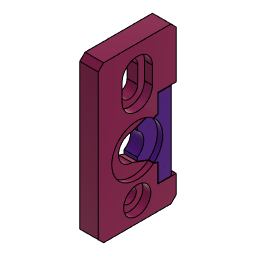
Rod_Holder_Hevo (Autodesk Fusion 360 design; units mm, degrees)
Autodesk Fusion 360 part; units mm, degrees
sketch "Sketch1" plane through (0, 0, 0) normal (1, 0, 0) x (0, 1, 0)
  circle A0 centre (0, 0) radius 5.1
  line L0 (-14.75, 35) -> (14.75, 35)
  line L1 (14.75, 35) -> (14.75, -24)
  line L2 (14.75, -24) -> (-14.75, -24)
  line L3 (-14.75, -24) -> (-14.75, 35)
  line L4 (0, 35) -> (0, -24)
  circle A1 centre (0, 25) radius 3.2
  circle A2 centre (0, 18.4) radius 3.15
  line L5 (0, 18.4) -> (3.15, 18.4) construction
  line L6 (0, 18.4) -> (-3.15, 18.4) construction
  line L7 (-3.15, 18.4) -> (-3.1999, 24.9757)
  line L8 (3.15, 18.4) -> (3.1999, 24.9757)
  arc A3 (5.75, 25) -> (-5.75, 25) centre (0, 25) ccw
  arc A4 (-5.75, 18.4) -> (5.75, 18.4) centre (0, 18.4) ccw
  line L9 (5.75, 18.4) -> (5.75, 25)
  line L10 (-5.75, 25) -> (-5.75, 18.4)
  circle A5 centre (0, -16.5) radius 2.65
  circle A6 centre (0, -16.5) radius 5.15
  line L11 (0, 5.1) -> (7.75, 8)
  line L12 (7.75, 8) -> (7.75, 15)
  line L13 (7.75, 15) -> (14.75, 15)
  line L14 (20, 0) -> (2.5, 0)
  line L15 (0, -5.1) -> (7.75, -8)
  line L16 (7.75, -8) -> (7.75, -15)
  line L17 (7.75, -15) -> (14.75, -15)
  dimension "d1" = 10.2
  dimension "d2" = 29.5
  dimension "d3" = 6.4
  dimension "d4" = 10
  dimension "d5" = 35
  dimension "d6" = 24
  dimension "d7" = 6.3
  dimension "d8" = 6.6
  dimension "d9" = 5.75
  dimension "d10" = 5.75
  dimension "d11" = 5.3
  dimension "d12" = 10.3
  dimension "d13" = 7.5
  dimension "d14" = 7
  dimension "d15" = 7
  dimension "d16" = 15
  constraint coincident A0.centre origin
  constraint horizontal L0
  constraint vertical L1
  constraint horizontal L2
  constraint vertical L3
  constraint midpoint L0 L4.start
  constraint midpoint L2 L4.end
  constraint coincident A0.centre L4
  constraint coincident L4 A1.centre
  constraint coincident L4 A2.centre
  constraint coincident A2.centre L5.start
  constraint coincident A2 L5.end
  constraint perpendicular L4 L5
  constraint coincident A2 L6.end
  constraint perpendicular L4 L6
  constraint coincident A1 L7.end
  constraint tangent A1 L7
  constraint coincident A1 L8.end
  constraint tangent A1 L8
  constraint coincident A1.centre A3.centre
  constraint tangent A3 L9
  constraint tangent A3 L10
  constraint vertical L9
  constraint vertical L10
  constraint coincident L4 A5.centre
  constraint concentric A5 A6
  constraint coincident L4 L11.start
  constraint coincident A0 L11.start
  constraint parallel L4 L12
  constraint coincident L1 L13.end
  constraint perpendicular L1 L13
  constraint symmetric L11.start L14 L15.start
  constraint symmetric L11.end L14 L15.end
  constraint symmetric L12.end L14 L16.end
  constraint symmetric L13.end L14 L17.end
  measures "d1" diameter of A0
  measures "d2" distance of L0.start L0.end
  measures "d3" diameter of A1
  measures "d4" distance of L0 A1.centre
  measures "d5" distance of A0.centre L0
  measures "d6" distance of A0.centre L2
  measures "d7" diameter of A2
  measures "d8" distance of A1.centre A2.centre
  measures "d9" radius of A3
  measures "d10" radius of A4
  measures "d11" diameter of A5
  measures "d12" diameter of A6
  measures "d13" distance of L4.end A5.centre
  measures "d14" distance of L12.end L13.end
  measures "d15" distance of L11.end L12.end
  measures "d16" distance of L13 L14
extrude "Extrude1" add sketch "Sketch1" along normal blind 7 contours A0 L0 L2 L3 L4 A3 A4 L10 A6 | L0 L1 L4 A3 A4 L9 L11 L12 L13 | L1 L2 L4 A6 L15 L16 L17 | L4 A1 A2 L7 A3 A4 L10 | L4 A1 A2 L8 A3 A4 L9 | L4 A5 A6 | L4 A5 A6 makes body 1
extrude "Extrude2" cut sketch "Sketch1" along normal up to surface (3 mm away) from surface at 4 contours L4 A1 A2 L7 A3 A4 L10 | L4 A1 A2 L8 A3 A4 L9 | L4 A5 A6 | L4 A5 A6 bodies 1
sketch "Sketch2" plane through (7, 0, 0) normal (1, 0, 0) x (0, 1, 0)
  arc A0 (-5.75, 18.4) -> (5.75, 18.4) centre (0, 18.4) ccw
  line L0 (-5.75, 18.4) -> (-5.75, 25)
  arc A1 (5.75, 25) -> (-5.75, 25) centre (0, 25) ccw
  line L1 (5.75, 25) -> (5.75, 18.4)
  circle A2 centre (0, -16.5) radius 5.15
  line L2 (0, 5.1) -> (7.75, 8)
  line L3 (7.75, 8) -> (7.75, 15)
  line L4 (7.75, 15) -> (14.75, 15)
  line L5 (14.75, 15) -> (14.75, 35)
  line L6 (14.75, 35) -> (-14.75, 35)
  line L7 (-14.75, 35) -> (-14.75, -24)
  line L8 (-14.75, -24) -> (14.75, -24)
  line L9 (14.75, -24) -> (14.75, -15)
  line L10 (14.75, -15) -> (7.75, -15)
  line L11 (7.75, -15) -> (7.75, -8)
  line L12 (7.75, -8) -> (0, -5.1)
  arc A3 (0, 5.1) -> (0, -5.1) centre (0, 0) ccw
  circle A4 centre (0, 0) radius 5.1
  constraint concentric A3 A4
  constraint coincident L2.start A4
sketch "Sketch1 (2)" plane through (7, 0, 0) normal (1, 0, 0) x (0, 1, 0) in component "Cap"
  arc A0 (-5.75, 18.4) -> (5.75, 18.4) centre (0, 18.4) ccw
  line L0 (-5.75, 18.4) -> (-5.75, 25)
  arc A1 (5.75, 25) -> (-5.75, 25) centre (0, 25) ccw
  line L1 (5.75, 25) -> (5.75, 18.4)
  circle A2 centre (0, -16.5) radius 5.15
  line L2 (0, 5.1) -> (7.75, 8)
  line L3 (7.75, 8) -> (7.75, 15)
  line L4 (7.75, 15) -> (14.75, 15)
  line L5 (14.75, 15) -> (14.75, 35)
  line L6 (14.75, 35) -> (-14.75, 35)
  line L7 (-14.75, 35) -> (-14.75, -24)
  line L8 (-14.75, -24) -> (14.75, -24)
  line L9 (14.75, -24) -> (14.75, -15)
  line L10 (14.75, -15) -> (7.75, -15)
  line L11 (7.75, -15) -> (7.75, -8)
  line L12 (7.75, -8) -> (0, -5.1)
  arc A3 (0, 5.1) -> (0, -5.1) centre (0, 0) ccw
  line L13 (14.9, 14.85) -> (14.9, 35.15)
  line L14 (14.9, 35.15) -> (-14.9, 35.15)
  line L15 (-14.9, 35.15) -> (-14.9, -24.15)
  line L16 (-14.9, -24.15) -> (14.9, -24.15)
  line L17 (14.9, -24.15) -> (14.9, -14.85)
  line L18 (14.9, -14.85) -> (7.9, -14.85)
  line L19 (7.9, -14.85) -> (7.9, -7.896)
  line L20 (7.9, -7.896) -> (0.0269, -4.9499)
  arc A4 (0.0269, 4.9499) -> (0.0269, -4.9499) centre (0, 0) ccw
  line L21 (0.0269, 4.9499) -> (7.9, 7.896)
  line L22 (7.9, 7.896) -> (7.9, 14.85)
  line L23 (7.9, 14.85) -> (14.9, 14.85)
  line L24 (2, 5.6882) -> (2, -5.6882)
  line L25 (12.9, 14.85) -> (12.9, -14.85)
  circle A5 centre (-0.5, 0) radius 5
  line L26 (0, 0) -> (-0.5, 0) construction
  dimension "d22" = 0.15
  dimension "d24" = 2
  dimension "d25" = 2
  dimension "d49" = 10
  dimension "d50" = 0.5
  constraint coincident L21 L24.start
  constraint coincident L20 L24.end
  constraint vertical L24
  constraint coincident L23 L25.start
  constraint coincident L18 L25.end
  constraint perpendicular L10 L25
  constraint coincident A3.centre A4.centre
  constraint coincident A5.centre L26.end
  constraint horizontal L26
  measures "d24" distance of A3.centre L24
  measures "d25" distance of L13.start L25
  measures "d49" diameter of A5
  measures "d50" distance of A3.centre A5.centre
extrude "Extrude1'" add sketch "Sketch1 (2)" against normal up to surface (7 mm away) separate body contours L18 L19 L20 L21 L22 L23 L24 L25 A5 makes body 2 in component "Cap"
sketch "Sketch2 (2)" plane through (0, 12.9, 0) normal (0, 1, 0) x (-1, 0, 0) in component "Cap"
  line L0 (0, -14.85) -> (0, 14.85)
  line L1 (0, 14.85) -> (-7, 14.85)
  line L2 (-7, 14.85) -> (-7, -14.85)
  line L3 (-7, -14.85) -> (0, -14.85)
  line L4 (-3.5, 14.85) -> (-3.5, -14.85) construction
  circle A0 centre (-3.5, 10.85) radius 1.65
  line L5 (0, 0) -> (-11, 0) construction
  circle A1 centre (-3.5, 10.85) radius 3.25
  circle A2 centre (-3.5, -10.85) radius 3.25
  circle A3 centre (-3.5, -10.85) radius 1.65
  dimension "d28" = 3.3
  dimension "d29" = 6.5
  dimension "d30" = 4
  constraint midpoint L1 L4.start
  constraint midpoint L3 L4.end
  constraint coincident L4 A0.centre
  constraint coincident L5.start origin
  constraint perpendicular L4 L5
  constraint concentric A0 A1
  constraint symmetric A0 L5 A3
  constraint symmetric L5 A1 A2
  measures "d28" diameter of A0
  measures "d29" diameter of A1
  measures "d30" distance of L1 A0.centre
extrude "Extrude3" cut sketch "Sketch2 (2)" against normal up to surface (9.15 mm away) contours A0 | A3 bodies 1
extrude "Extrude2'" cut sketch "Sketch2 (2)" against normal up to surface (9.15 mm away) contours A0 | A3 bodies 2 in component "Cap"
sketch "Sketch3" plane through (-0.2586, 7.75, 0.0748) normal (0, 1, 0) x (-1, 0, 0) in component "Cap"
  circle A0 centre (-3.7586, 10.7752) radius 1.65
  line L0 (-0.2586, 7.9252) -> (-0.2586, 14.9252)
  line L1 (-0.2586, 14.9252) -> (-7.2586, 14.9252)
  line L2 (-7.2586, 14.9252) -> (-7.2586, 7.9252)
  line L3 (-7.2586, 7.9252) -> (-0.2586, 7.9252)
sketch "Sketch3 (2)" plane through (0, 7.75, 0) normal (0, 1, 0) x (-1, 0, 0)
  circle A0 centre (-3.5, 10.85) radius 1.65
  line L0 (0, 8) -> (0, 15)
  line L1 (0, 15) -> (-7, 15)
  line L2 (-7, 15) -> (-7, 8)
  line L3 (-7, 8) -> (0, 8)
  circle A1 centre (-3.5, 10.85) radius 2.05
  circle A2 centre (-3.5, -10.85) radius 1.65
  line L4 (0, -15) -> (0, -8)
  line L5 (0, -8) -> (-7, -8)
  line L6 (-7, -8) -> (-7, -15)
  line L7 (-7, -15) -> (0, -15)
  circle A3 centre (-3.5, -10.85) radius 2.05
  dimension "d35" = 4.1
  dimension "d36" = 4.1
  constraint concentric A0 A1
  constraint concentric A2 A3
  measures "d35" diameter of A1
  measures "d36" diameter of A3
extrude "Extrude4" cut sketch "Sketch3 (2)" against normal blind 4 contours A1 | A3 bodies 1
sketch "Sketch4" plane through (0.2586, 12.9, -0.0748) normal (0, 1, 0) x (-1, 0, 0)
  circle A0 centre (-3.2414, -10.7752) radius 1.65
  circle A1 centre (-3.2414, 10.9248) radius 1.65
  line L0 (0.2586, -14.7752) -> (0.2586, 14.9248)
  line L1 (0.2586, 14.9248) -> (-6.7414, 14.9248)
  line L2 (-6.7414, 14.9248) -> (-6.7414, -14.7752)
  line L3 (-6.7414, -14.7752) -> (0.2586, -14.7752)
  circle A2 centre (-3.2414, 10.9248) radius 3.25
  circle A3 centre (-3.2414, -10.7752) radius 3.25
  dimension "d39" = 6.5
  dimension "d40" = 6.5
  constraint concentric A1 A2
  constraint concentric A0 A3
  measures "d39" diameter of A2
  measures "d40" diameter of A3
extrude "Extrude3'" cut sketch "Sketch4" against normal blind 2.5 contours A2 | A3 bodies 2 in component "Cap"
chamfer "Chamfer1" distance 2 angle 45 4 edges at (3.5, -14.75, 35) (3.5, 14.75, 35) (3.5, -14.75, -24) (3.5, 14.75, -24) on bodies 1
sketch "Sketch5" plane through (7, 0, 0) normal (1, 0, 0) x (0, 1, 0)
  line L0 (12.75, -24) -> (14.75, -22)
  line L1 (14.75, -22) -> (14.75, -15)
  line L2 (14.75, -15) -> (7.75, -15)
  line L3 (7.75, -15) -> (7.75, -8)
  line L4 (7.75, -8) -> (0, -5.1)
  arc A0 (0, 5.1) -> (0, -5.1) centre (0, 0) ccw
  line L5 (0, 5.1) -> (7.75, 8)
  line L6 (7.75, 8) -> (7.75, 15)
  line L7 (7.75, 15) -> (14.75, 15)
  line L8 (14.75, 15) -> (14.75, 33)
  line L9 (14.75, 33) -> (12.75, 35)
  line L10 (12.75, 35) -> (-12.75, 35)
  line L11 (-12.75, 35) -> (-14.75, 33)
  line L12 (-14.75, 33) -> (-14.75, -22)
  line L13 (-14.75, -22) -> (-12.75, -24)
  line L14 (-12.75, -24) -> (12.75, -24)
  arc A1 (-5.75, 18.4) -> (5.75, 18.4) centre (0, 18.4) ccw
  line L15 (-5.75, 18.4) -> (-5.75, 25)
  arc A2 (5.75, 25) -> (-5.75, 25) centre (0, 25) ccw
  line L16 (5.75, 25) -> (5.75, 18.4)
  circle A3 centre (0, -16.5) radius 5.15
  circle A4 centre (0, 0) radius 9.65
  dimension "d44" = 19.3
  constraint concentric A0 A4
  measures "d44" diameter of A4
extrude "Extrude5" cut sketch "Sketch5" against normal blind 2 contours L4 A0 L5 A4 | L4 A0 L5 A4 bodies 1
extrude "Extrude4'" cut sketch "Sketch5" against normal blind 2 contours L4 A0 L5 A4 | L4 A0 L5 A4 bodies 2 in component "Cap"
component "Cap" placed x (1, 0, 0) y (0, 1, 0) z (0, 0, 1) at (0, 0, 0)
equation "d9 = ( 11.5 / 2 ) * 1 mm"
equation "d10 = ( 11.5 / 2 ) * 1 mm"
